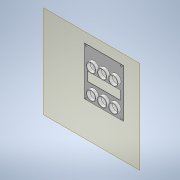
# Autodesk Inventor part: vial holder
Saved by Autodesk Inventor 2022 (Build 260153000, 153)
## iProperties
Created: 2022-05-04
Part Number: vial holder
Material: Generic
Document SubType Name: Modeling
Designer: efred
Density: 1 g/cm^3
Appearance: Default
Author: efred
Autodesk Inventor part; units mm, degrees
ref_plane "YZ Plane" through (0, 0, 0) normal (1, 0, 0) x (0, 1, 0)
ref_plane "XZ Plane" through (0, 0, 0) normal (0, 1, 0) x (-1, 0, 0)
ref_plane "XY Plane" through (0, 0, 0) normal (0, 0, 1) x (1, 0, 0)
ref_plane "Work Plane1" through (0, 0, 0) normal (0, 0, 1) x (1, 0, 0)
sketch "Sketch1" plane through (0, 0, 0) normal (0, 0, 1) x (1, 0, 0)
  circle A0 centre (41.875, 20.01) radius 13.75 projected
  circle A1 centre (4.875, 20.01) radius 13.75 projected
  circle A2 centre (-32.125, 20.01) radius 13.75 projected
  circle A3 centre (41.875, 100.01) radius 13.75 projected
  circle A4 centre (4.875, 100.01) radius 13.75 projected
  circle A5 centre (-32.125, 100.01) radius 13.75 projected
  line L0 (65, 0.01) -> (65, 140.01) projected
  line L1 (65, 140.01) -> (-65, 140.01) projected
  line L2 (-65, 140.01) -> (-65, 0.01) projected
  line L3 (-65, 0.01) -> (65, 0.01) projected
  line L4 (65, -9.99) -> (65, 150.01) projected
  line L5 (65, 150.01) -> (-65, 150.01) projected
  line L6 (-65, 150.01) -> (-65, -9.99) projected
  line L7 (-65, -9.99) -> (65, -9.99) projected
  circle A6 centre (-59, -5.99) radius 2.9 projected
  circle A7 centre (-59, 146.01) radius 2.9 projected
  circle A8 centre (59, 146.01) radius 2.9 projected
  circle A9 centre (59, -5.99) radius 2.9 projected
  circle A10 centre (41.875, 20.01) radius 13.95
  circle A11 centre (4.875, 20.01) radius 13.95
  circle A12 centre (-32.125, 20.01) radius 13.95
  circle A13 centre (41.875, 100.01) radius 13.95
  circle A14 centre (4.875, 100.01) radius 13.95
  circle A15 centre (-32.125, 100.01) radius 13.95
  line L8 (-65, 140.01) -> (65, 140.01)
  line L9 (65, 140.01) -> (65, 0.01)
  line L10 (65, 0.01) -> (-65, 0.01)
  line L11 (-65, 0.01) -> (-65, 140.01)
  line L12 (55, 45.01) -> (-55, 45.01)
  line L13 (-55, 45.01) -> (-55, 75.01)
  line L14 (-55, 75.01) -> (55, 75.01)
  line L15 (55, 75.01) -> (55, 45.01)
  point P0 (0, 0)
  point P1 (65, 0.01)
  point P2 (-65, 0.01)
  point P3 (-65, 140.01)
  point P4 (65, 140.01)
  dimension "d0" = 0.2
  dimension "d1" = 0.2
  dimension "d2" = 0.2
  dimension "d3" = 0.2
  dimension "d4" = 0.2
  dimension "d5" = 0.2
  dimension "d6" = 0
  dimension "d17" = 25
  dimension "d18" = 25
  dimension "d19" = 10
  dimension "d20" = 10
  constraints: 16 end point, 6 centre point, 2 parallel, 1 horizontal, 1 perpendicular, 3 other
  measures "d0" radial gap between concentric circles of A0 A10
  measures "d1" radial gap between concentric circles of A1 A11
  measures "d2" radial gap between concentric circles of A2 A12
  measures "d3" radial gap between concentric circles of A3 A13
  measures "d4" radial gap between concentric circles of A4 A14
  measures "d5" radial gap between concentric circles of A5 A15
  measures "d6" distance between parallel lines of L1 L8
  measures "d17" distance from line of A1.centre L12
  measures "d18" distance from line of A4.centre L14
  measures "d19" distance between parallel lines of L0 L15
  measures "d20" distance between parallel lines of L6 L13
extrude "Extrusion1" add sketch "Sketch1" along normal blind 1 contours L3 L2 L1 L0 | L4 L7 L6 L3 | L1 L6 L5 L4
sketch "Sketch2" plane through (0, 0, 1) normal (0, 0, 1) x (1, 0, 0)
  line L0 (65, -9.99) -> (65, 150.01) projected
  line L1 (-65, 150.01) -> (-65, -9.99) projected
  circle A0 centre (-32.125, 100.01) radius 13.95 projected
  circle A1 centre (4.875, 100.01) radius 13.95 projected
  circle A2 centre (41.875, 100.01) radius 13.95 projected
  circle A3 centre (-32.125, 20.01) radius 13.95 projected
  circle A4 centre (4.875, 20.01) radius 13.95 projected
  circle A5 centre (41.875, 20.01) radius 13.95 projected
  circle A6 centre (41.875, 20.01) radius 15.95
  circle A7 centre (4.875, 20.01) radius 15.95
  circle A8 centre (-32.125, 20.01) radius 15.95
  circle A9 centre (-32.125, 100.01) radius 15.95
  circle A10 centre (4.875, 100.01) radius 15.95
  circle A11 centre (41.875, 100.01) radius 15.95
  line L2 (65, 150.01) -> (-65, 150.01) projected
  line L3 (-65, -9.99) -> (65, -9.99) projected
  point P0 (0, 0)
  dimension "d9" = 2
  dimension "d10" = 2
  dimension "d11" = 2
  dimension "d12" = 2
  dimension "d13" = 2
  dimension "d14" = 2
  constraints: 6 centre point
  measures "d9" radial gap between concentric circles of A5 A6
  measures "d10" radial gap between concentric circles of A4 A7
  measures "d11" radial gap between concentric circles of A3 A8
  measures "d12" radial gap between concentric circles of A0 A9
  measures "d13" radial gap between concentric circles of A1 A10
  measures "d14" radial gap between concentric circles of A2 A11
extrude "Extrusion2" add sketch "Sketch2" along normal blind 10 contours A6 | A7 | A8 | A9 | A10 | A11
body "Solid1"
